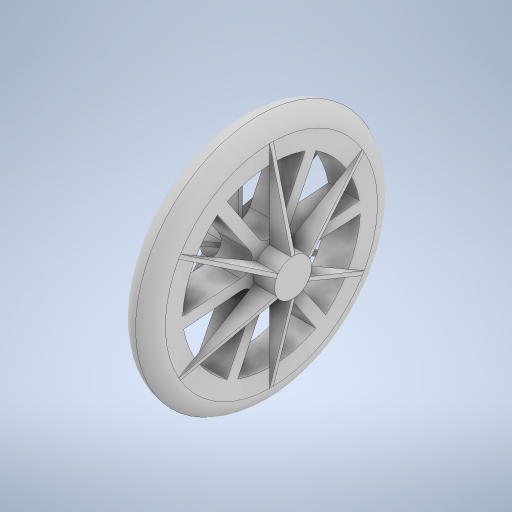
# Autodesk Inventor part: zfront wheel
Saved by Autodesk Inventor 2023 (Build 270158000, 158)
## iProperties
Created: 2023-11-07
Part Number: zfront wheel
Material: Generic
Document SubType Name: Modeling
Designer: HP
Density: 1 g/cm^3
Appearance: Default
Author: HP
Autodesk Inventor part; units mm, degrees
ref_plane "YZ Plane" through (0, 0, 0) normal (1, 0, 0) x (0, 1, 0)
ref_plane "XZ Plane" through (0, 0, 0) normal (0, 1, 0) x (-1, 0, 0)
ref_plane "XY Plane" through (0, 0, 0) normal (0, 0, 1) x (1, 0, 0)
sketch "Sketch1" plane through (0, 0, 0) normal (1, 0, 0) x (0, 1, 0)
  circle A0 centre (0, 0) radius 100
  dimension "d2" = 200
  constraints: 1 centre point, 1 coincident
  measures "d2" diameter of A0
extrude "Extrusion1" add sketch "Sketch1" along normal mid plane 25
sketch "Sketch2" plane through (12.5, 0, 0) normal (1, 0, 0) x (0, 0, -1)
  circle A0 centre (0, 0) radius 15
  dimension "d3" = 30
  constraints: 1 centre point, 1 coincident
  measures "d3" diameter of A0
extrude "Extrusion2" add sketch "Sketch2" along normal blind 17.5 and the other way blind 42.5
sketch "Sketch3" plane through (12.5, 0, 0) normal (1, 0, 0) x (0, 0, -1)
  line L0 (0, 0) -> (35.3822, 71.7503)
  line L1 (0, 0) -> (79.8286, 5.2333)
  arc A0 (79.8286, 5.2333) -> (35.3822, 71.7503) centre (0, 0) ccw
  line L2 (15.0568, 20.2371) -> (36.0061, 62.2334)
  line L3 (24.8068, 5.8055) -> (71.1164, 9.5295)
  arc A1 (15.0568, 20.2371) -> (24.8068, 5.8055) centre (24.0053, 15.7733) ccw
  arc A2 (71.1164, 9.5295) -> (36.0061, 62.2334) centre (-7.5807, -4.8501) ccw
  dimension "d8" = 80
  dimension "d10" = 80
  dimension "d12" = 60
  dimension "d14" = 10
  dimension "d15" = 80
  constraints: 8 end point, 6 point on circle, 3 centre point, 2 tangent
  measures "d8" distance of L0.start L0.end
  measures "d10" distance of L0.start L1.end
  measures "d12" angle of L1 L0
  measures "d14" radius of A1
  measures "d15" radius of A2
extrude "Extrusion3" cut sketch "Sketch3" against normal blind 25 contours L2 A2 L3 A1
pattern_circular "Circular Pattern1" count 6 over 360 about axis through (12.5, 0, 0) along (1, 0, 0) of "Extrusion3"
fillet "Fillet1" radius 15 1 edges at (-12.5, -100, 0)
fillet "Fillet2" radius 15 1 edges at (12.5, -100, 0)
sketch "Sketch4" plane through (0, 0, 0) normal (0, 0, 1) x (1, 0, 0)
  line L0 (30, -15) -> (30, 15) projected
  line L1 (12.5, 85.8579) -> (12.5, -85.8579) projected
  line L2 (30, 15) -> (12.5, 85.8579)
  line L3 (12.5, 85.8579) -> (12.5, 15)
  line L4 (30, 15) -> (12.5, 15)
  line L5 (12.5, 18.5806) -> (-12.5, 18.5806) projected
  point P0 (0, 0)
  constraints: 6 end point, 1 parallel, 1 point on line
extrude "Extrusion4" add sketch "Sketch4" along normal mid plane 3
pattern_circular "Circular Pattern2" count 6 over 360 about axis through (12.5, 0, 0) along (1, 0, 0) of "Extrusion4"
mirror "Mirror1" about plane through (0, 0, 0) normal (1, 0, 0) of "Extrusion4", "Circular Pattern2"
ref_plane "Work Plane1" through (0, 0, 0) normal (1, 0, 0) x (0, 1, 0)
body "Solid1"
